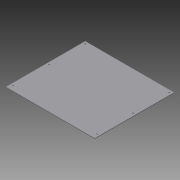
# Autodesk Inventor part: polycarb bottom
Saved by Autodesk Inventor 2015 SP1 (Build 190203100, 203)
## iProperties
Created: 2015-01-16
Part Number: polycarb bottom
Material: Generic
Document SubType Name: Modeling
Designer: Jarod
Density: 1 g/cm^3
Appearance: Default
Author: Jarod
Autodesk Inventor part; units mm, degrees
ref_plane "YZ Plane" through (0, 0, 0) normal (1, 0, 0) x (0, 1, 0)
ref_plane "XZ Plane" through (0, 0, 0) normal (0, 1, 0) x (-1, 0, 0)
ref_plane "XY Plane" through (0, 0, 0) normal (0, 0, 1) x (1, 0, 0)
sketch "Sketch1" plane through (0, 0, 0) normal (0, 1, 0) x (-1, 0, 0)
  line L0 (0, 0) -> (-469.9, 0)
  line L1 (-469.9, 0) -> (-469.9, 419.1)
  line L2 (-469.9, 419.1) -> (0, 419.1)
  line L3 (0, 419.1) -> (0, 0)
  dimension "d0" = 469.9
  dimension "d1" = 419.1
  constraints: 8 end point, 2 parallel, 1 horizontal, 1 perpendicular
  measures "d0" distance of L1.end L2.end
  measures "d1" distance of L0.end L1.end
extrude "Extrusion1" add sketch "Sketch1" along normal blind 3.175
sketch "Sketch2" plane through (0, 3.175, 0) normal (0, 1, 0) x (1, 0, 0)
  line L0 (469.9, 0) -> (0, 0) projected
  line L1 (0, 0) -> (0, -419.1) projected
  line L2 (0, -419.1) -> (469.9, -419.1) projected
  line L3 (469.9, -419.1) -> (469.9, 0) projected
  point P0 (12.7, -12.7)
  point P1 (12.7, -203.2)
  point P2 (12.7, -393.7)
  point P3 (457.2, -12.7)
  point P4 (457.2, -203.2)
  point P5 (457.2, -393.7)
  dimension "d4" = 12.7
  dimension "d5" = 12.7
  dimension "d6" = 12.7
  dimension "d7" = 12.7
  dimension "d8" = 12.7
  dimension "d11" = 12.7
  dimension "d12" = 12.7
  dimension "d13" = 12.7
  dimension "d14" = 203.2
  dimension "d15" = 203.2
  dimension "d16" = 25.4
  dimension "d17" = 25.4
  measures "d4" distance from line of L1 point (12.7, -12.7)
  measures "d5" distance from line of L0 point (12.7, -12.7)
  measures "d6" distance from line of L0 point (457.2, -12.7)
  measures "d7" distance from line of L3 point (457.2, -12.7)
  measures "d8" distance from line of L3 point (457.2, -393.7)
  measures "d11" distance from line of L1 point (12.7, -393.7)
  measures "d12" distance from line of L1 point (12.7, -203.2)
  measures "d13" distance from line of L3 point (457.2, -203.2)
  measures "d14" distance from line of L0 point (12.7, -203.2)
  measures "d15" distance from line of L0 point (457.2, -203.2)
  measures "d16" distance from line of L2 point (12.7, -393.7)
  measures "d17" distance from line of L2 point (457.2, -393.7)
hole "Hole1" at (12.7, 3.175, 12.7) at (12.7, 3.175, 203.2) at (12.7, 3.175, 393.7) at (457.2, 3.175, 12.7) at (457.2, 3.175, 203.2) at (457.2, 3.175, 393.7) direction (0, -1, 0) diameter 6.35 end through all
body "Solid1"
